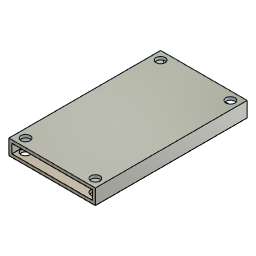
Ass v5 (Autodesk Fusion 360 archive; units mm, degrees)
design "Cellule chauffante"
Autodesk Fusion 360 part; units mm, degrees
sketch "Esquisse1" plane through (0, 0, 0) normal (0, 1, 0) x (1, 0, 0)
  line L0 (0, 0) -> (28.5, 0)
  line L1 (28.5, 0) -> (28.5, -50)
  line L2 (28.5, -50) -> (0, -50)
  line L3 (0, -50) -> (0, 0)
  circle A0 centre (2.75, -2.75) radius 1.5
  circle A1 centre (25.75, -2.75) radius 1.5
  circle A2 centre (2.75, -47.25) radius 1.5
  circle A3 centre (25.75, -47.25) radius 1.5
  dimension "d1" = 28.5
  dimension "d2" = 50
  dimension "d3" = 3
  dimension "d4" = 3
  dimension "d5" = 3
  dimension "d6" = 3
  dimension "d7" = 2.75
  dimension "d8" = 2.75
  dimension "d9" = 2.75
  dimension "d10" = 2.75
  dimension "d11" = 2.75
  dimension "d12" = 2.75
  dimension "d13" = 2.75
  dimension "d14" = 2.75
  constraint horizontal L0
  constraint vertical L1
  constraint horizontal L2
  constraint vertical L3
  constraint coincident L0.start L3.end
  measures "d1" distance of L0.start L0.end
  measures "d2" distance of L0.end L1.end
  measures "d3" diameter of A2
  measures "d4" diameter of A3
  measures "d5" diameter of A1
  measures "d6" diameter of A0
  measures "d7" distance of L0 A0.centre
  measures "d8" distance of L3 A0.centre
  measures "d9" distance of L0 A1.centre
  measures "d10" distance of L1 A1.centre
  measures "d11" distance of L3 A2.centre
  measures "d12" distance of L2 A2.centre
  measures "d13" distance of L2 A3.centre
  measures "d14" distance of L1 A3.centre
extrude "Extrusion1" add sketch "Esquisse1" along normal blind 5
sketch "Esquisse2" plane through (0, 0, 0) normal (0, 0, -1) x (-1, 0, 0)
  line L0 (-28.5, 0) -> (0, 0)
  line L1 (0, 0) -> (0, 5)
  line L2 (0, 5) -> (-28.5, 5)
  line L3 (-28.5, 5) -> (-28.5, 0)
  line L4 (-27.5, 4) -> (-1, 4)
  line L5 (-1, 4) -> (-1, 1)
  line L6 (-1, 1) -> (-27.5, 1)
  line L7 (-27.5, 1) -> (-27.5, 4)
  dimension "d17" = 1
  dimension "d18" = 1
  dimension "d19" = 1
  dimension "d20" = 1
  constraint horizontal L4
  constraint vertical L5
  constraint horizontal L6
  constraint vertical L7
  measures "d17" distance of L2 L4
  measures "d18" distance of L3 L7
  measures "d19" distance of L0 L6
  measures "d20" distance of L1 L5
extrude "Extrusion2" cut sketch "Esquisse2" against normal blind 71 contours L4 L5 L6 L7
sketch "Esquisse3" plane through (0, 5, 0) normal (0, 1, 0) x (-1, 0, 0)
  circle A0 centre (-2.75, 2.75) radius 1.5
  circle A1 centre (-2.75, 47.25) radius 1.5
  circle A2 centre (-25.75, 2.75) radius 1.5
  circle A3 centre (-25.75, 47.25) radius 1.5
  line L0 (0, 50) -> (-28.5, 50)
  line L1 (-28.5, 50) -> (-28.5, 0)
  line L2 (-28.5, 0) -> (0, 0)
  line L3 (0, 0) -> (0, 50)

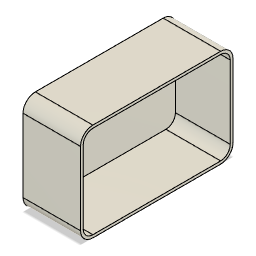
design "support inf"
Autodesk Fusion 360 part; units mm, degrees
sketch "Esquisse1" plane through (0, 0, 0) normal (1, 0, 0) x (0, 0, -1)
  line L0 (166.9054, -107.1527) -> (-0.0946, -107.1527)
  circle A0 centre (13.4054, -93.6527) radius 13.5
  line L1 (-0.0946, -107.1527) -> (-0.0946, -0.1527)
  circle A1 centre (13.4054, -13.6527) radius 13.5
  line L2 (-0.0946, -0.1527) -> (166.9054, -0.1527)
  circle A2 centre (153.4054, -13.6527) radius 13.5
  line L3 (166.9054, -0.1527) -> (166.9054, -107.1527)
  circle A3 centre (153.4054, -93.6527) radius 13.5
  dimension "d44" = 107
  dimension "d45" = 167
  dimension "d24" = 27
  dimension "d25" = 27
  dimension "d26" = 27
  dimension "d27" = 27
  constraint horizontal L2
  constraint vertical L3
  constraint horizontal L0
  constraint vertical L1
  measures "d44" distance of L2.end L0.start
  measures "d45" distance of L2.end L1.end
  measures "d24" diameter of A2
  measures "d25" diameter of A1
  measures "d26" diameter of A3
  measures "d27" diameter of A0
extrude "Extrusion3" add sketch "Esquisse1" along normal blind 3 contours L0 A0 L1 A1 L2 A2 L3 A3 | A3 | A0 | A2 | A1
sketch "Esquisse3" plane through (3, 0, 0) normal (1, 0, 0) x (0, 0, -1)
  arc A0 (13.4054, -0.1527) -> (-0.0946, -13.6527) centre (13.4054, -13.6527) ccw
  line L0 (-0.0946, -13.6527) -> (-0.0946, -93.6527)
  arc A1 (-0.0946, -93.6527) -> (13.4054, -107.1527) centre (13.4054, -93.6527) ccw
  line L1 (13.4054, -107.1527) -> (153.4054, -107.1527)
  arc A2 (153.4054, -107.1527) -> (166.9054, -93.6527) centre (153.4054, -93.6527) ccw
  line L2 (166.9054, -93.6527) -> (166.9054, -13.6527)
  arc A3 (166.9054, -13.6527) -> (153.4054, -0.1527) centre (153.4054, -13.6527) ccw
  line L3 (153.4054, -0.1527) -> (13.4054, -0.1527)
  line L4 (13.4054, -0.1527) -> (13.4054, -107.1527)
  line L5 (-0.0946, -13.6527) -> (166.9054, -13.6527)
  line L6 (153.4054, -0.1527) -> (153.4054, -107.1527)
  line L7 (166.9054, -93.6527) -> (-0.0946, -93.6527)
  line L8 (13.4054, -3.1527) -> (153.4054, -3.1527)
  line L9 (163.9054, -13.6527) -> (163.9054, -93.6527)
  line L10 (153.4054, -104.1527) -> (13.4054, -104.1527)
  line L11 (2.9054, -93.6527) -> (2.9054, -13.6527)
  line L12 (-0.0946, -0.1527) -> (166.9054, -0.1527)
  line L13 (-0.0946, -107.1527) -> (-0.0946, -0.1527)
  line L14 (166.9054, -107.1527) -> (-0.0946, -107.1527)
  line L15 (166.9054, -0.1527) -> (166.9054, -107.1527)
  arc A4 (13.4054, -3.1527) -> (2.9054, -13.6527) centre (13.4054, -13.6527) ccw
  arc A5 (163.9054, -13.6527) -> (153.4054, -3.1527) centre (153.4054, -13.6527) ccw
  arc A6 (2.9054, -93.6527) -> (13.4054, -104.1527) centre (13.4054, -93.6527) ccw
  arc A7 (153.4054, -104.1527) -> (163.9054, -93.6527) centre (153.4054, -93.6527) ccw
  dimension "d52" = 3
  dimension "d53" = 3
  dimension "d54" = 3
  dimension "d55" = 3
  constraint coincident A0.start L3.end
  constraint coincident A1.end L1.start
  constraint coincident A0.end L0.start
  constraint coincident L2.end A3.start
  constraint coincident A3.end L3.start
  constraint coincident L1.end A2.start
  constraint coincident A2.end L2.start
  constraint coincident L0.end A1.start
  constraint coincident L4 L8.start
  constraint coincident L6 L8.end
  constraint perpendicular L6 L8
  constraint coincident L5 L9.start
  constraint coincident L7 L9.end
  constraint perpendicular L7 L9
  constraint coincident L6 L10.start
  constraint coincident L4 L10.end
  constraint perpendicular L4 L10
  constraint coincident L7 L11.start
  constraint coincident L5 L11.end
  constraint perpendicular L5 L11
  constraint coincident A0.centre A4.centre
  constraint coincident A1.centre A6.centre
  measures "d52" distance of L8 L12
  measures "d53" distance of L11 L13
  measures "d54" distance of L10 L14
  measures "d55" distance of L9 L15
extrude "Extrusion4" add sketch "Esquisse3" along normal blind 60 contours A0 L4 L5 A4 | L3 L4 L6 L8 L12 | L0 L5 L7 L11 L13 | A3 L5 L6 A5 | A1 L4 L7 A6 | L2 L5 L7 L9 L15 | L1 L4 L6 L10 L14 | A2 L6 L7 A7
equation "d10 = largEntrePied + diaPiedBois"
equation "d11 = longEntrePied + diaPiedBois"
equation "d12 = diaPiedBois"
equation "d13 = diaExtPiedBois / 2"
equation "d14 = diaExtPiedBois / 2"
equation "d15 = diaPiedBois"
equation "d16 = diaPiedBois"
equation "d17 = diaPiedBois"
equation "d18 = diaExtPiedBois / 2"
equation "d44 = largEntrePied + diaExtPiedBois"
equation "d45 = longEntrePied + diaExtPiedBois"
equation "d24 = diaPiedBois + 5 mm"
equation "d25 = diaPiedBois + 5 mm"
equation "d26 = diaPiedBois + 5 mm"
equation "d27 = diaPiedBois + 5 mm"

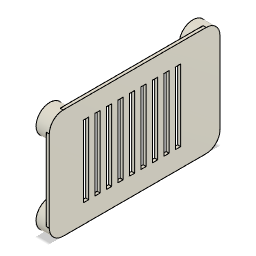
design "support dip"
Autodesk Fusion 360 part; units mm, degrees
sketch "Esquisse1" plane through (0, 0, 0) normal (1, 0, 0) x (0, 0, -1)
  line L0 (-0.0946, -0.1527) -> (166.9054, -0.1527)
  line L1 (166.9054, -0.1527) -> (166.9054, -107.1527)
  line L2 (166.9054, -107.1527) -> (-0.0946, -107.1527)
  line L3 (-0.0946, -107.1527) -> (-0.0946, -0.1527)
  circle A0 centre (153.4054, -13.6527) radius 11
  circle A1 centre (13.4054, -13.6527) radius 11
  circle A2 centre (13.4054, -93.6527) radius 11
  circle A3 centre (153.4054, -93.6527) radius 11
  circle A4 centre (153.4054, -13.6527) radius 13.5
  circle A5 centre (153.4054, -93.6527) radius 13.5
  circle A6 centre (13.4054, -93.6527) radius 13.5
  circle A7 centre (13.4054, -13.6527) radius 13.5
  dimension "d10" = 107
  dimension "d11" = 167
  dimension "d12" = 22
  dimension "d13" = 13.5
  dimension "d14" = 13.5
  dimension "d15" = 22
  dimension "d16" = 22
  dimension "d17" = 22
  dimension "d18" = 13.5
  dimension "d19" = 13.5
  dimension "d20" = 13.5
  dimension "d21" = 13.5
  dimension "d22" = 13.5
  dimension "d23" = 13.5
  dimension "d24" = 27
  dimension "d25" = 27
  dimension "d26" = 27
  dimension "d27" = 27
  constraint horizontal L0
  constraint vertical L1
  constraint horizontal L2
  constraint vertical L3
  constraint concentric A0 A4
  constraint concentric A3 A5
  constraint concentric A2 A6
  constraint concentric A1 A7
  measures "d10" distance of L0.end L1.end
  measures "d11" distance of L0.start L0.end
  measures "d12" diameter of A0
  measures "d13" distance of L0 A0.centre
  measures "d14" distance of L1 A0.centre
  measures "d15" diameter of A1
  measures "d16" diameter of A2
  measures "d17" diameter of A3
  measures "d18" distance of L0 A1.centre
  measures "d19" distance of L3 A1.centre
  measures "d20" distance of L3 A2.centre
  measures "d21" distance of L2 A2.centre
  measures "d22" distance of L2 A3.centre
  measures "d23" distance of L1 A3.centre
  measures "d24" diameter of A4
  measures "d25" diameter of A7
  measures "d26" diameter of A5
  measures "d27" diameter of A6
extrude "Extrusion1" add sketch "Esquisse1" along normal blind 3 contours L0 L1 L2 L3 A4 A5 A6 A7 | A7 | A4 | A6 | A5 | A0 | A1 | A2 | A3
extrude "Extrusion2" add sketch "Esquisse1" against normal blind 10 contours A7 | A4 | A6 | A5
sketch "Esquisse3" plane through (0, 0, 0) normal (-1, 0, 0) x (0, 0, 1)
  arc A0 (-166.9054, -13.6527) -> (-153.4054, -0.1527) centre (-153.4054, -13.6527) ccw
  line L0 (-166.9054, -13.6527) -> (-166.9054, -93.6527)
  arc A1 (-153.4054, -107.1527) -> (-166.9054, -93.6527) centre (-153.4054, -93.6527) ccw
  line L1 (-153.4054, -107.1527) -> (-13.4054, -107.1527)
  arc A2 (0.0946, -93.6527) -> (-13.4054, -107.1527) centre (-13.4054, -93.6527) ccw
  line L2 (0.0946, -93.6527) -> (0.0946, -13.6527)
  arc A3 (-13.4054, -0.1527) -> (0.0946, -13.6527) centre (-13.4054, -13.6527) ccw
  line L3 (-13.4054, -0.1527) -> (-153.4054, -0.1527)
  line L4 (-78.4054, -88.6527) -> (-83.4054, -88.6527)
  line L5 (-83.4054, -88.6527) -> (-83.4054, -18.6527)
  line L6 (-83.4054, -18.6527) -> (-78.4054, -18.6527)
  line L7 (-78.4054, -18.6527) -> (-78.4054, -88.6527)
  line L8 (-72.1554, -88.6527) -> (-72.1554, -18.6527)
  line L9 (-67.1554, -88.6527) -> (-72.1554, -88.6527)
  line L10 (-67.1554, -18.6527) -> (-67.1554, -88.6527)
  line L11 (-72.1554, -18.6527) -> (-67.1554, -18.6527)
  line L12 (-60.9054, -88.6527) -> (-60.9054, -18.6527)
  line L13 (-55.9054, -88.6527) -> (-60.9054, -88.6527)
  line L14 (-55.9054, -18.6527) -> (-55.9054, -88.6527)
  line L15 (-60.9054, -18.6527) -> (-55.9054, -18.6527)
  line L16 (-49.6554, -88.6527) -> (-49.6554, -18.6527)
  line L17 (-44.6554, -88.6527) -> (-49.6554, -88.6527)
  line L18 (-44.6554, -18.6527) -> (-44.6554, -88.6527)
  line L19 (-49.6554, -18.6527) -> (-44.6554, -18.6527)
  line L20 (-38.4054, -88.6527) -> (-38.4054, -18.6527)
  line L21 (-33.4054, -88.6527) -> (-38.4054, -88.6527)
  line L22 (-33.4054, -18.6527) -> (-33.4054, -88.6527)
  line L23 (-38.4054, -18.6527) -> (-33.4054, -18.6527)
  line L24 (-94.6554, -88.6527) -> (-94.6554, -18.6527)
  line L25 (-89.6554, -18.6527) -> (-89.6554, -88.6527)
  line L26 (-89.6554, -88.6527) -> (-94.6554, -88.6527)
  line L27 (-94.6554, -18.6527) -> (-89.6554, -18.6527)
  line L28 (-105.9054, -88.6527) -> (-105.9054, -18.6527)
  line L29 (-100.9054, -18.6527) -> (-100.9054, -88.6527)
  line L30 (-100.9054, -88.6527) -> (-105.9054, -88.6527)
  line L31 (-105.9054, -18.6527) -> (-100.9054, -18.6527)
  line L32 (-117.1554, -88.6527) -> (-117.1554, -18.6527)
  line L33 (-112.1554, -18.6527) -> (-112.1554, -88.6527)
  line L34 (-112.1554, -88.6527) -> (-117.1554, -88.6527)
  line L35 (-117.1554, -18.6527) -> (-112.1554, -18.6527)
  line L36 (-128.4054, -88.6527) -> (-128.4054, -18.6527)
  line L37 (-123.4054, -18.6527) -> (-123.4054, -88.6527)
  line L38 (-123.4054, -88.6527) -> (-128.4054, -88.6527)
  line L39 (-128.4054, -18.6527) -> (-123.4054, -18.6527)
  dimension "d35" = 5
  dimension "d36" = 70
  dimension "d37" = 83.5
  dimension "d38" = 18.5
  dimension "d41" = 45
  dimension "d42" = 0
  dimension "d45" = -45
  dimension "d46" = 0
  constraint horizontal L4
  constraint vertical L5
  constraint horizontal L6
  constraint vertical L7
  measures "d35" distance of L4.start L4.end
  measures "d36" distance of L4.end L5.end
  measures "d37" distance of L0 L5
  measures "d38" distance of L1 L4
extrude "Extrusion3" cut sketch "Esquisse3" against normal blind 25 contours L4 L5 L6 L7 | L8 L9 L10 L11 | L12 L13 L14 L15 | L16 L17 L18 L19 | L20 L21 L22 L23 | L24 L25 L26 L27 | L28 L29 L30 L31 | L32 L33 L34 L35 | L36 L37 L38 L39
equation "diaPiedBois = 22 mm"
equation "longEntrePied = 140 mm"
equation "largEntrePied = 80 mm"
equation "d10 = largEntrePied + diaExtPiedBois"
equation "d11 = longEntrePied + diaExtPiedBois"
equation "d12 = diaPiedBois"
equation "d13 = diaExtPiedBois / 2"
equation "d14 = diaExtPiedBois / 2"
equation "d15 = diaPiedBois"
equation "d16 = diaPiedBois"
equation "d17 = diaPiedBois"
equation "d18 = diaExtPiedBois / 2"
equation "d19 = diaExtPiedBois / 2"
equation "d20 = diaExtPiedBois / 2"
equation "d21 = diaExtPiedBois / 2"
equation "d22 = diaExtPiedBois / 2"
equation "d23 = diaExtPiedBois / 2"
equation "d24 = diaPiedBois + 5 mm"
equation "d25 = diaPiedBois + 5 mm"
equation "d26 = diaPiedBois + 5 mm"
equation "d27 = diaPiedBois + 5 mm"
equation "diaExtPiedBois = diaPiedBois + 5 mm"
equation "d29 = epPlaqueHaut"
equation "d31 = -hautSupportPiedBois"
equation "epPlaqueHaut = 3 mm"
equation "hautSupportPiedBois = 10 mm"
equation "d37 = ( longEntrePied + diaExtPiedBois ) / 2"
equation "d38 = ( largEntrePied + diaExtPiedBois ) / 2 - ( 70 / 2 ) * 1 mm"

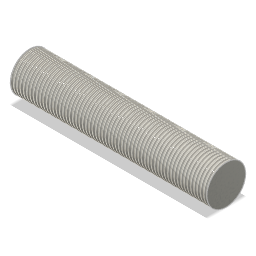
design "Support disipateur"
Autodesk Fusion 360 part; units mm, degrees
sketch "Esquisse1" plane through (0, 0, 0) normal (1, 0, 0) x (0, 0, -1)
  circle A0 centre (0, 0) radius 3
  dimension "d1" = 6
  constraint coincident A0.centre origin
  measures "d1" diameter of A0
extrude "Extrusion1" add sketch "Esquisse1" along normal blind 30
thread "Filetage1" "ISO Metric profile 6.0 M6x0.5 6g" major diameter 5.927 minor diameter 5.3505 pitch 0.5 angle 60 resizes the face on face at (20, -0.2987, -2.9851)

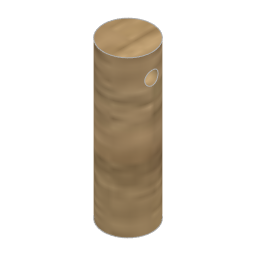
design "Pilier"
Autodesk Fusion 360 part; units mm, degrees
sketch "Esquisse1" plane through (0, 0, 0) normal (0, 1, 0) x (1, 0, 0)
  circle A0 centre (0, 0) radius 10.925
  dimension "d1" = 21.85
  constraint coincident A0.centre origin
  measures "d1" diameter of A0
extrude "Extrusion1" add sketch "Esquisse1" along normal blind 70
sketch "Esquisse2" plane through (0, 0, 0) normal (1, 0, 0) x (0, 0, -1)
  line L0 (0, 70) -> (0, 60)
  circle A0 centre (0, 60) radius 3
  dimension "d4" = 10
  dimension "d5" = 6
  constraint vertical L0
  constraint coincident L0.end A0.centre
  measures "d4" distance of L0.start L0.end
  measures "d5" diameter of A0
extrude "Extrusion2" cut sketch "Esquisse2" along normal blind 17
